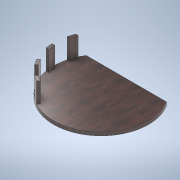
# Autodesk Inventor part: Nest-ver2-1111-2021
Saved by Autodesk Inventor 2021 (Build 250183000, 183)
## iProperties
Created: 2021-03-02
Part Number: Nest-ver2-1111-2021
Material: Generic
Document SubType Name: Modeling
Designer: CMurray
Density: 1 g/cm^3
Appearance: White Oak - Wild Berries
Author: CMurray
Autodesk Inventor part; units mm, degrees
ref_plane "YZ Plane" through (0, 0, 0) normal (1, 0, 0) x (0, 1, 0)
ref_plane "XZ Plane" through (0, 0, 0) normal (0, 1, 0) x (-1, 0, 0)
ref_plane "XY Plane" through (0, 0, 0) normal (0, 0, 1) x (1, 0, 0)
sketch "Sketch2" plane through (0, 0, 0) normal (0, 1, 0) x (-1, 0, 0)
  arc A0 (762, -479.9355) -> (-762, -479.9355) centre (0, 0) ccw
  line L0 (900.5455, 0) -> (762, 0)
  line L1 (762, -479.9355) -> (-762, -479.9355)
  dimension "d8" = 1524
  constraints: 4 end point, 3 point on circle, 1 centre point, 1 coincident, 1 horizontal
  measures "d8" distance of L1.start L1.end
extrude "Extrusion1" add sketch "Sketch2" along normal blind 63.5
sketch "Sketch4" plane through (0, 63.5, 0) normal (0, 1, 0) x (1, 0, 0)
  arc A0 (-762, 479.9355) -> (762, 479.9355) centre (0, 0) ccw
  line L0 (762, 479.9355) -> (-762, 479.9355) projected
  arc A1 (-762, 479.9355) -> (762, 479.9355) centre (0, 0) ccw projected
  line L1 (-762, 479.9355) -> (762, 479.9355)
  line L2 (-790.3185, 352.9355) -> (-828.5038, 352.9355)
  line L3 (-790.3185, 352.9355) -> (-790.3185, 225.9355)
  line L4 (-790.3185, 225.9355) -> (-871.7427, 225.9355)
  dimension "d15" = 127
  constraints: 8 end point, 4 point on circle, 2 horizontal, 1 centre point, 1 coincident, 1 perpendicular, 1 vertical
  measures "d15" distance of L2.start L3.end
extrude "Extrusion4" add sketch "Sketch4" along normal blind 381 contours L2 L3 L4 A0
sketch "Sketch5" plane through (0, 63.5, 0) normal (0, 1, 0) x (1, 0, 0)
  line L0 (-790.3185, 225.9355) -> (-871.7427, 225.9355) projected
  arc A0 (-762, 479.9355) -> (762, 479.9355) centre (0, 0) ccw
  arc A1 (-762, 479.9355) -> (762, 479.9355) centre (0, 0) ccw projected
  arc A2 (-871.7427, 225.9355) -> (762, 479.9355) centre (0, 0) ccw projected
  line L1 (-871.7427, 225.9355) -> (-790.3185, 225.9355) projected
  line L2 (-790.3185, 225.9355) -> (-790.3185, -28.0645)
  line L3 (-790.3185, -28.0645) -> (-900.108, -28.0645)
  line L4 (-790.3185, -28.0645) -> (-790.3185, -155.0645)
  line L5 (-790.3185, -155.0645) -> (-887.0948, -155.0645)
  line L6 (762, 479.9355) -> (-762, 479.9355) projected
  line L7 (762, 479.9355) -> (-762, 479.9355)
  dimension "d23" = 254
  dimension "d24" = 127
  constraints: 10 end point, 4 point on circle, 2 perpendicular, 1 centre point, 1 coincident, 1 horizontal, 1 point on line, 1 vertical
  measures "d23" distance of L0.start L2.end
  measures "d24" distance of L2.end L4.end
extrude "Extrusion6" add sketch "Sketch5" along normal blind 381 contours L4 L5 A0 L3
sketch "Sketch6" plane through (0, 63.5, 0) normal (0, 1, 0) x (1, 0, 0)
  arc A0 (-762, 479.9355) -> (762, 479.9355) centre (0, 0) ccw
  line L0 (762, 479.9355) -> (-762, 479.9355) projected
  arc A1 (-762, 479.9355) -> (762, 479.9355) centre (0, 0) ccw projected
  line L1 (-762, 479.9355) -> (762, 479.9355)
  line L2 (-790.3185, -155.0645) -> (-790.3185, -431.7161)
  arc A2 (-887.0948, -155.0645) -> (762, 479.9355) centre (0, 0) ccw projected
  line L3 (-790.3185, -431.7161) -> (-688.5633, -355.7235)
  line L4 (-688.5633, -355.7235) -> (-612.5707, -457.4787)
  line L5 (-612.5707, -457.4787) -> (-721.537, -538.8567)
  dimension "d27" = 127
  dimension "d28" = 127
  dimension "d29" = 127
  dimension "d30" = 90
  dimension "d31" = 90
  constraints: 10 end point, 4 point on circle, 1 centre point, 1 coincident, 1 horizontal, 1 vertical
  measures "d27" distance of L2.end L3.end
  measures "d28" distance from line of A0.centre L3
  measures "d29" distance of L3.end L4.end
  measures "d30" angle of L4 L3
  measures "d31" angle of L5 L4
extrude "Extrusion7" add sketch "Sketch6" along normal blind 381 contours L3 L4 L5 A0
sketch "Sketch7" plane through (0, 63.5, 0) normal (0, 1, 0) x (1, 0, 0)
  arc A0 (-762, 479.9355) -> (762, 479.9355) centre (0, 0) ccw
  line L0 (-762, 479.9355) -> (762, 479.9355)
  arc A1 (-721.537, -538.8567) -> (762, 479.9355) centre (0, 0) ccw projected
  line L1 (-540.1977, -716.7108) -> (-439.217, -613.7513)
  line L2 (-439.217, -613.7513) -> (-348.5473, -702.6783)
  line L3 (-348.5473, -702.6783) -> (-433.5292, -789.3254)
  line L4 (-540.1977, -716.7108) -> (-542.3554, -718.9108)
  arc A2 (-762, 479.9355) -> (762, 479.9355) centre (0, 0) ccw projected
  dimension "d34" = 254
  dimension "d35" = 127
  dimension "d36" = 90
  constraints: 10 end point, 4 point on circle, 1 centre point, 1 coincident, 1 perpendicular
  measures "d34" distance of A1.start L1.start
  measures "d35" distance of L1.end L2.end
  measures "d36" angle of L3 L2
extrude "Extrusion8" add sketch "Sketch7" along normal blind 381 contours L4 L1 L2 L3 A0
sketch "Sketch8" plane through (0, 63.5, 0) normal (0, 1, 0) x (1, 0, 0)
  arc A0 (-762, 479.9355) -> (762, 479.9355) centre (0, 0) ccw
  line L0 (762, 479.9355) -> (-762, 479.9355) projected
  line L1 (762, 479.9355) -> (-762, 479.9355)
  arc A1 (-733.4235, 429.1355) -> (733.4235, 429.1355) centre (0, 0) ccw
  line L2 (-733.4235, 429.1355) -> (733.4235, 429.1355)
  dimension "d39" = 50.8
  constraints: 4 end point, 4 point on circle, 2 centre point, 1 coincident, 1 collinear, 1 other
  measures "d39" radial gap between concentric circles of A0 A1
extrude "Extrusion9" cut sketch "Sketch8" along normal blind 381 contours L2 A1
body "Solid1"
